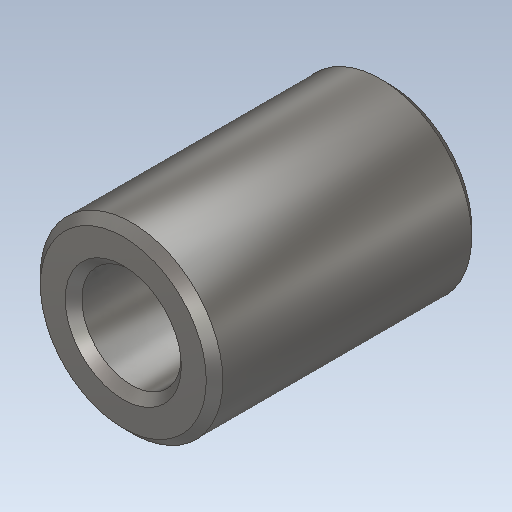
# Autodesk Inventor part: Cartesian1_LinearBearing
Saved by Autodesk Inventor 2020 (Build 240168000, 168)
## iProperties
Created: 2020-02-29
Part Number: Cartesian1_LinearBearing
Material: Stal, stopowa
Document SubType Name: Modeling
Designer: invin
Density: 7.73 g/cm^3
Appearance: Częściowo polerowana
Mass: 65.2282 g
Surface Area: 38.2698 cm^2
Volume: 8.43832 cm^3
Author: invin
Autodesk Inventor part; units mm, degrees
ref_plane "YZ Plane" through (0, 0, 0) normal (1, 0, 0) x (0, 1, 0)
ref_plane "XZ Plane" through (0, 0, 0) normal (0, 1, 0) x (-1, 0, 0)
ref_plane "XY Plane" through (0, 0, 0) normal (0, 0, 1) x (1, 0, 0)
sketch "Szkic1" plane through (0, 0, 0) normal (0, 0, 1) x (1, 0, 0)
  circle A0 centre (0, 0) radius 6
  circle A1 centre (0, 0) radius 11
  dimension "d0" = 12
  dimension "d1" = 22
  constraints: 2 centre point, 2 coincident
  measures "d0" diameter of A0
  measures "d1" diameter of A1
extrude "Wyciągnięcie proste1" add sketch "Szkic1" along normal blind 32
chamfer "Faza1" distance 1 angle 45 4 edges at (-11, 0, 32) (-6, 0, 32) (-6, 0, 0) (-11, 0, 0)
